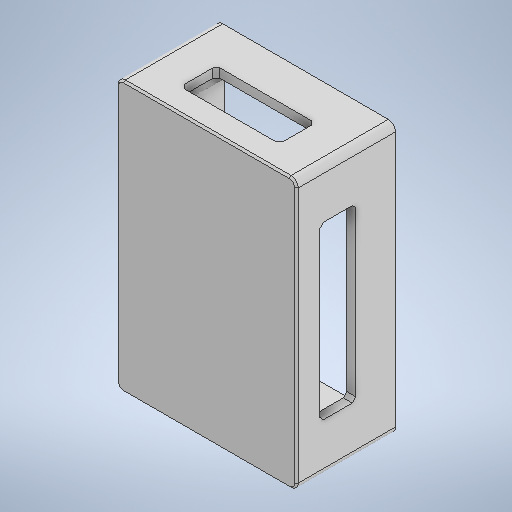
# Autodesk Inventor part: PCB_Case
Saved by Autodesk Inventor 2025.3 (Build 293356000, 356)
## iProperties
Created: 2025-11-23
Part Number: PCB_Case
Material: Generic
Document SubType Name: Modeling
Designer: Wula
Density: 1 g/cm^3
Appearance: Default
Author: Wula
Autodesk Inventor part; units mm, degrees
ref_plane "YZ Plane" through (0, 0, 0) normal (1, 0, 0) x (0, 1, 0)
ref_plane "XZ Plane" through (0, 0, 0) normal (0, 1, 0) x (-1, 0, 0)
ref_plane "XY Plane" through (0, 0, 0) normal (0, 0, 1) x (1, 0, 0)
sketch "Sketch1" plane through (0, 0, 0) normal (0, 1, 0) x (-1, 0, 0)
  line L0 (-50, 75) -> (50, 75)
  line L1 (50, 75) -> (50, -75)
  line L2 (50, -75) -> (-50, -75)
  line L3 (-50, -75) -> (-50, 75)
  line L4 (-50, 75) -> (50, -75) construction
  line L5 (50, 75) -> (-50, -75) construction
  point P0 (0, 0)
  dimension "d0" = 150
  dimension "d1" = 100
  constraints: 12 end point, 2 midpoint, 2 parallel, 1 horizontal, 1 perpendicular
  measures "d0" distance of L0.end L1.end
  measures "d1" distance of L0.start L0.end
extrude "Extrusion1" add sketch "Sketch1" along normal blind 55
shell "Shell1" thickness 5 removed faces 1 at (16.6667, 55, 25)
sketch "Sketch2" plane through (0, 55, 0) normal (0, 1, 0) x (1, 0, 0)
  line L0 (-45, -70) -> (-45, 70) projected
  line L1 (-50, 75) -> (-50, -75) projected
  arc A0 (-28, -75) -> (-50, -53) centre (-50, -75) ccw
  line L2 (-50, 75) -> (-50, -75) projected
  line L3 (-50, -53) -> (-50, -75)
  line L4 (-50, -75) -> (-28, -75)
  line L5 (-50, -75) -> (50, -75) projected
  line L6 (0, -75) -> (0, 75)
  line L7 (50, 75) -> (-50, 75) projected
  line L8 (-50, 0) -> (45, 0)
  arc A1 (-50, 53) -> (-28, 75) centre (-50, 75) ccw
  line L9 (-50, 53) -> (-50, 75)
  line L10 (-50, 75) -> (-28, 75)
  line L11 (0, 75) -> (0, -75)
  arc A2 (50, -53) -> (28, -75) centre (50, -75) ccw
  line L12 (50, -53) -> (50, -75)
  line L13 (50, -75) -> (28, -75)
  arc A3 (28, 75) -> (50, 53) centre (50, 75) ccw
  line L14 (50, 53) -> (50, 75)
  line L15 (50, 75) -> (28, 75)
  point P0 (0, 0)
  point P1 (45, -70)
  point P2 (45, 70)
  point P3 (28, 75)
  point P4 (28, -75)
  point P5 (-28, 75)
  point P6 (-50, 53)
  dimension "d6" = 22
  constraints: 22 end point, 10 symmetric about line, 8 point on circle, 4 centre point, 3 midpoint, 1 horizontal, 1 perpendicular, 1 point on line, 1 vertical, 3 other
  measures "d6" distance of L1.end L3.start
extrude "Extrusion2" add sketch "Sketch2" against normal blind 55 contours A0 L4 L1 | A1 L1 L7 | A2 L12 L5 | L14 A3 L7
sketch "Sketch3" plane through (-28.5757, 5, -70) normal (0, 1, 0) x (1, 0, 0)
  line L0 (62.8657, -115.72) -> (-5.7143, -115.72) construction
  line L1 (-5.7143, -115.72) -> (-5.7143, -24.28) construction
  line L2 (-5.7143, -24.28) -> (62.8657, -24.28) construction
  line L3 (62.8657, -24.28) -> (62.8657, -115.72) construction
  line L4 (62.8657, -115.72) -> (-5.7143, -24.28) construction
  line L5 (-5.7143, -115.72) -> (62.8657, -24.28) construction
  circle A0 centre (-5.7143, -115.72) radius 4
  circle A1 centre (-5.7143, -115.72) radius 2
  circle A2 centre (-5.7143, -24.28) radius 4
  circle A3 centre (-5.7143, -24.28) radius 2
  circle A4 centre (62.8657, -24.28) radius 4
  circle A5 centre (62.8657, -24.28) radius 2
  circle A6 centre (62.8657, -115.72) radius 4
  circle A7 centre (62.8657, -115.72) radius 2
  circle A8 centre (1.5679, -103.22) radius 4
  circle A9 centre (1.5679, -103.22) radius 2
  point P0 (28.5757, -70)
  dimension "d12" = 91.44
  dimension "d13" = 68.58
  dimension "d14" = 8
  dimension "d15" = 4
  dimension "d16" = 8
  dimension "d17" = 4
  dimension "d18" = 8
  dimension "d19" = 4
  dimension "d20" = 8
  dimension "d21" = 4
  dimension "d22" = 8
  dimension "d23" = 4
  constraints: 13 coincident, 12 end point, 10 centre point, 2 midpoint, 2 parallel, 1 horizontal, 1 perpendicular
  measures "d12" distance of L0.end L1.end
  measures "d13" distance of L0.start L0.end
  measures "d14" diameter of A0
  measures "d15" diameter of A1
  measures "d16" diameter of A2
  measures "d17" diameter of A3
  measures "d18" diameter of A4
  measures "d19" diameter of A5
  measures "d20" diameter of A6
  measures "d21" diameter of A7
  measures "d22" diameter of A8
  measures "d23" diameter of A9
extrude "Extrusion3" add sketch "Sketch3" along normal blind 5 contours A0 | A2 | A4 | A6
sketch "Sketch6" plane through (50, 0, -75) normal (0, 0, -1) x (-1, 0, 0)
  line L0 (0, 0) -> (100, 0) projected
  line L1 (78.5757, 55) -> (78.5757, 5) projected
  line L2 (21.4243, 5) -> (21.4243, 55) projected
  line L3 (24.5, 13) -> (75.5, 13)
  line L4 (77.5, 15) -> (77.5, 31)
  line L5 (75.5, 33) -> (24.5, 33)
  line L6 (22.5, 31) -> (22.5, 15)
  line L7 (22.5, 13) -> (77.5, 33) construction
  line L8 (77.5, 13) -> (22.5, 33) construction
  line L9 (21.4243, 55) -> (78.5757, 55) projected
  line L10 (50, 55) -> (50, 0) construction
  line L11 (24.5, 33) -> (22.5, 31)
  line L12 (75.5, 33) -> (77.5, 31)
  line L13 (22.5, 15) -> (24.5, 13)
  line L14 (77.5, 15) -> (75.5, 13)
  point P0 (50, 23)
  dimension "d47" = 55
  dimension "d48" = 20
  dimension "d49" = 23
  dimension "d58" = 2
  dimension "d59" = 2
  dimension "d60" = 2
  dimension "d61" = 2
  dimension "d62" = 2
  dimension "d63" = 2
  dimension "d64" = 2
  dimension "d65" = 2
  constraints: 22 end point, 9 point on line, 3 midpoint, 2 parallel, 2 perpendicular, 1 horizontal
  measures "d47" distance of L7.end L8.end
  measures "d48" distance of L8.start L7.end
  measures "d49" distance from line of L0 point (50, 23)
  measures "d58" distance of L5.end L8.end
  measures "d59" distance of L6.start L8.end
  measures "d60" distance of L5.start L7.end
  measures "d61" distance of L4.end L7.end
  measures "d62" distance of L6.end L7.start
  measures "d63" distance of L3.start L7.start
  measures "d64" distance of L4.start L8.start
  measures "d65" distance of L3.end L8.start
extrude "Extrusion4" cut sketch "Sketch6" against normal through all
sketch "Sketch7" plane through (50, 0, 75) normal (1, 0, 0) x (0, 0, -1)
  line L0 (75, 0) -> (75, 54.6826)
  line L1 (29.5, 13) -> (120.5, 13)
  line L2 (122.5, 15) -> (122.5, 31)
  line L3 (120.5, 33) -> (29.5, 33)
  line L4 (27.5, 31) -> (27.5, 15)
  line L5 (27.5, 13) -> (122.5, 33) construction
  line L6 (122.5, 13) -> (27.5, 33) construction
  line L7 (0, 0) -> (150, 0) projected
  line L8 (29.5, 33) -> (27.5, 31)
  line L9 (27.5, 15) -> (29.5, 13)
  line L10 (120.5, 13) -> (122.5, 15)
  line L11 (122.5, 31) -> (120.5, 33)
  point P0 (75, 23)
  dimension "d76" = 95
  dimension "d77" = 20
  dimension "d78" = 23
  dimension "d79" = 2
  dimension "d80" = 2
  dimension "d81" = 2
  dimension "d82" = 2
  dimension "d83" = 2
  dimension "d84" = 2
  dimension "d85" = 2
  dimension "d86" = 2
  constraints: 22 end point, 9 point on line, 2 midpoint, 2 parallel, 1 horizontal, 1 perpendicular, 1 vertical
  measures "d76" distance of L6.end L5.end
  measures "d77" distance of L5.end L6.start
  measures "d78" distance from line of L7 point (75, 23)
  measures "d79" distance of L3.end L6.end
  measures "d80" distance of L4.start L6.end
  measures "d81" distance of L4.end L5.start
  measures "d82" distance of L1.start L5.start
  measures "d83" distance of L1.end L6.start
  measures "d84" distance of L2.start L6.start
  measures "d85" distance of L2.end L5.end
  measures "d86" distance of L3.start L5.end
extrude "Extrusion5" cut sketch "Sketch7" against normal through all
sketch "Sketch8" plane through (0, 55, 0) normal (0, 1, 0) x (1, 0, 0)
  line L0 (-44.2093, -69.2093) -> (-45.75, -66.5407)
  line L1 (-45.75, -66.5407) -> (-45.75, -63.4593)
  line L2 (-45.75, -63.4593) -> (-44.2093, -60.7907)
  line L3 (-44.2093, -60.7907) -> (-41.5407, -59.25)
  line L4 (-41.5407, -59.25) -> (-38.4593, -59.25)
  line L5 (-38.4593, -59.25) -> (-35.7907, -60.7907)
  line L6 (-35.7907, -60.7907) -> (-34.25, -63.4593)
  line L7 (-34.25, -63.4593) -> (-34.25, -66.5407)
  line L8 (-34.25, -66.5407) -> (-35.7907, -69.2093)
  line L9 (-35.7907, -69.2093) -> (-38.4593, -70.75)
  line L10 (-38.4593, -70.75) -> (-41.5407, -70.75)
  line L11 (-41.5407, -70.75) -> (-44.2093, -69.2093)
  line L12 (-50, 75) -> (-50, -75) projected
  line L13 (-50, -75) -> (50, -75) projected
  line L14 (-41.5407, 70.75) -> (-38.4593, 70.75)
  line L15 (-38.4593, 70.75) -> (-35.7907, 69.2093)
  line L16 (-44.2093, 69.2093) -> (-41.5407, 70.75)
  line L17 (-35.7907, 69.2093) -> (-34.25, 66.5407)
  line L18 (-45.75, 63.4593) -> (-45.75, 66.5407)
  line L19 (-34.25, 66.5407) -> (-34.25, 63.4593)
  line L20 (-34.25, 63.4593) -> (-35.7907, 60.7907)
  line L21 (-44.2093, 60.7907) -> (-45.75, 63.4593)
  line L22 (-35.7907, 60.7907) -> (-38.4593, 59.25)
  line L23 (-38.4593, 59.25) -> (-41.5407, 59.25)
  line L24 (-41.5407, 59.25) -> (-44.2093, 60.7907)
  line L25 (-45.75, 66.5407) -> (-44.2093, 69.2093)
  line L26 (38.4593, -59.25) -> (41.5407, -59.25)
  line L27 (41.5407, -59.25) -> (44.2093, -60.7907)
  line L28 (35.7907, -60.7907) -> (38.4593, -59.25)
  line L29 (44.2093, -60.7907) -> (45.75, -63.4593)
  line L30 (34.25, -66.5407) -> (34.25, -63.4593)
  line L31 (45.75, -63.4593) -> (45.75, -66.5407)
  line L32 (45.75, -66.5407) -> (44.2093, -69.2093)
  line L33 (35.7907, -69.2093) -> (34.25, -66.5407)
  line L34 (44.2093, -69.2093) -> (41.5407, -70.75)
  line L35 (41.5407, -70.75) -> (38.4593, -70.75)
  line L36 (38.4593, -70.75) -> (35.7907, -69.2093)
  line L37 (34.25, -63.4593) -> (35.7907, -60.7907)
  line L38 (38.4593, 70.75) -> (41.5407, 70.75)
  line L39 (41.5407, 70.75) -> (44.2093, 69.2093)
  line L40 (35.7907, 69.2093) -> (38.4593, 70.75)
  line L41 (44.2093, 69.2093) -> (45.75, 66.5407)
  line L42 (34.25, 63.4593) -> (34.25, 66.5407)
  line L43 (45.75, 66.5407) -> (45.75, 63.4593)
  line L44 (45.75, 63.4593) -> (44.2093, 60.7907)
  line L45 (35.7907, 60.7907) -> (34.25, 63.4593)
  line L46 (44.2093, 60.7907) -> (41.5407, 59.25)
  line L47 (41.5407, 59.25) -> (38.4593, 59.25)
  line L48 (38.4593, 59.25) -> (35.7907, 60.7907)
  line L49 (34.25, 66.5407) -> (35.7907, 69.2093)
  point P0 (0, 0)
  point P1 (-40, -65)
  point P2 (-50, 71)
  point P3 (-50, -71)
  point P4 (-46, -75)
  point P5 (46, -75)
  point P6 (-40, 65)
  point P7 (40, -65)
  point P8 (40, 65)
  dimension "d103" = 11.5
  dimension "d104" = 10
  dimension "d105" = 10
  dimension "d108" = 130
  dimension "d111" = 80
  constraints: 96 end point, 2 horizontal, 1 vertical, 100 other
  measures "d103" distance between parallel lines of L4 L10
  measures "d104" distance from line of L12 point (-40, -65)
  measures "d105" distance from line of L13 point (-40, -65)
  measures "d108" distance of L3.end L14.start
  measures "d111" distance of L3.end L26.start
extrude "Extrusion6" cut sketch "Sketch8" against normal blind 5.5
sketch "Sketch9" plane through (0, 49.5, 0) normal (0, 1, 0) x (1, 0, 0)
  circle A0 centre (-40, -65) radius 3.25
  line L0 (-50, 75) -> (-50, -75) projected
  line L1 (-50, -75) -> (50, -75) projected
  circle A1 centre (-40, 65) radius 3.25
  circle A2 centre (40, -65) radius 3.25
  circle A3 centre (40, 65) radius 3.25
  point P0 (0, 0)
  point P1 (-50, 71)
  point P2 (-50, -71)
  point P3 (-46, -75)
  point P4 (46, -75)
  dimension "d116" = 6.5
  dimension "d117" = 10
  dimension "d118" = 10
  dimension "d121" = 130
  dimension "d124" = 80
  constraints: 4 centre point, 1 horizontal, 1 vertical, 6 other
  measures "d116" diameter of A0
  measures "d117" distance from line of L0 A0.centre
  measures "d118" distance from line of A0.centre L1
  measures "d121" distance of A0.centre A1.centre
  measures "d124" distance of A0.centre A2.centre
extrude "Extrusion7" cut sketch "Sketch9" against normal blind 40
fillet "Fillet1" radius 4 4 edges at (50, 27.5, 75) (-50, 27.5, 75) (50, 27.5, -75) (-50, 27.5, -75)
chamfer "Chamfer3" distance 1 angle 45 8 edges at (0, 0, 75) (48.8284, 0, 73.8284) (50, 0, 0) (48.8284, 0, -73.8284) (0, 0, -75) (-48.8284, 0, -73.8284) (-50, 0, 0) (-48.8284, 0, 73.8284)
equation "\"d59\" = d58"
equation "\"d60\" = d58"
equation "\"d61\" = d60"
equation "\"d62\" = d58"
equation "\"d63\" = d62"
equation "\"d64\" = d58"
equation "\"d65\" = d64"
equation "\"d80\" = d79"
equation "\"d81\" = d79"
equation "\"d82\" = d81"
equation "\"d83\" = d79"
equation "\"d84\" = d83"
equation "\"d85\" = d79"
equation "\"d86\" = d85"
body "Solid1"
